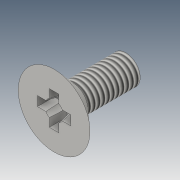
# Autodesk Inventor part: Parafuso do Escudo
Saved by Autodesk Inventor 2016 (Build 200138000, 138)
## iProperties
Created: 2018-12-10
Part Number: Parafuso do Escudo
Material: Generic
Document SubType Name: Modeling
Designer: Pedro Mendonça
Density: 1 g/cm^3
Appearance: Default
Author: Pedro Mendonça
Autodesk Inventor part; units mm, degrees
ref_plane "YZ Plane" through (0, 0, 0) normal (1, 0, 0) x (0, 1, 0)
ref_plane "XZ Plane" through (0, 0, 0) normal (0, 1, 0) x (-1, 0, 0)
sketch "Sketch1" plane through (0, 0, 0) normal (1, 0, 0) x (0, 1, 0)
  circle A0 centre (0, 0) radius 1.5
  dimension "d0" = 3
  constraints: 1 centre point, 1 coincident
  measures "d0" diameter of A0
extrude "Extrusion1" add sketch "Sketch1" against normal blind 5.5
ref_plane "Work Plane1" through (2, 0, 0) normal (1, 0, 0) x (0, 0, -1)
sketch "Sketch2" plane through (2, 0, 0) normal (1, 0, 0) x (0, 0, -1)
  circle A0 centre (0, 0) radius 3.75
  dimension "d4" = 7.5
  constraints: 1 centre point, 1 coincident
  measures "d4" diameter of A0
loft "Loft1" add profiles "Sketch2" section 1 edges at (0, -1.5, 0)
sketch "Sketch3" plane through (2, 0, 0) normal (1, 0, 0) x (0, 0, -1)
  line L0 (-0.5, -1.75) -> (0.5, -1.75)
  line L1 (0.5, 1.75) -> (-0.5, 1.75)
  line L2 (1.75, -0.5) -> (1.75, 0.5)
  line L3 (-1.75, 0.5) -> (-1.75, -0.5)
  line L4 (0.5, -1.75) -> (0.5, -0.866)
  line L5 (0.5, 0.866) -> (0.5, 1.75)
  line L6 (-1.75, -0.5) -> (-0.866, -0.5)
  line L7 (0.866, -0.5) -> (1.75, -0.5)
  arc A0 (0.5, -0.866) -> (0.866, -0.5) centre (0, 0) ccw
  line L8 (1.75, 0.5) -> (0.866, 0.5)
  line L9 (-0.866, 0.5) -> (-1.75, 0.5)
  line L10 (-0.5, 1.75) -> (-0.5, 0.866)
  line L11 (-0.5, -0.866) -> (-0.5, -1.75)
  arc A1 (0.866, 0.5) -> (0.5, 0.866) centre (0, 0) ccw
  arc A2 (-0.5, 0.866) -> (-0.866, 0.5) centre (0, 0) ccw
  arc A3 (-0.866, -0.5) -> (-0.5, -0.866) centre (0, 0) ccw
  dimension "d9" = 1
  dimension "d10" = 3.5
  dimension "d11" = 1
  dimension "d12" = 3.5
  constraints: 24 end point, 10 parallel, 8 point on circle, 4 centre point, 4 perpendicular, 1 horizontal
  measures "d9" distance of L1.end L1.start
  measures "d10" distance of L1.start L0.end
  measures "d11" distance of L3.end L3.start
  measures "d12" distance of L3.start L2.end
extrude "Extrusion2" cut sketch "Sketch3" against normal blind 1.5 draft -10
thread "Thread1" size "M3x0.5" class "6g" standard "ANSI Metric M Profile" full length
body "Solid1"
